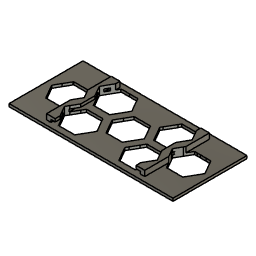
huine_solar_controller_mount (Autodesk Fusion 360 design; units mm, degrees)
Autodesk Fusion 360 part; units mm, degrees
sketch "Sketch1" plane through (0, 0, 0) normal (0, 0, 1) x (1, 0, 0)
  line L0 (0, 0) -> (-152, 0)
  line L1 (-152, 0) -> (-152, 68.58)
  line L2 (-152, 68.58) -> (0, 68.58)
  line L3 (0, 68.58) -> (0, 0)
  dimension "d1" = 152
  dimension "d2" = 68.58
  constraint horizontal L0
  constraint vertical L1
  constraint horizontal L2
  constraint vertical L3
  constraint coincident L0.start L3.end
  measures "d1" distance of L0.start L0.end
  measures "d2" distance of L0.start L2.end
extrude "Extrude1" add sketch "Sketch1" along normal blind 2.5
sketch "Sketch2" plane through (0, 0, 2.5) normal (0, 0, 1) x (-1, 0, 0)
  line L0 (0, -68.58) -> (152, -68.58)
  line L1 (152, -68.58) -> (152, 0)
  line L2 (152, 0) -> (0, 0)
  line L3 (0, 0) -> (0, -68.58)
  line L4 (76, -68.58) -> (76, 0) construction
  line L5 (152, -34.29) -> (0, -34.29) construction
  line L6 (117, -11.54) -> (35, -11.54) construction
  line L7 (35, -11.54) -> (35, -57.04) construction
  line L8 (35, -57.04) -> (117, -57.04) construction
  line L9 (117, -57.04) -> (117, -11.54) construction
  line L10 (117, -11.54) -> (35, -57.04) construction
  line L11 (35, -11.54) -> (117, -57.04) construction
  line L12 (113.5, -4.29) -> (120.5, -4.29)
  line L13 (120.5, -4.29) -> (120.5, -64.29)
  line L14 (120.5, -64.29) -> (113.5, -64.29)
  line L15 (113.5, -64.29) -> (113.5, -4.29)
  line L16 (113.5, -4.29) -> (120.5, -64.29) construction
  line L17 (120.5, -4.29) -> (113.5, -64.29) construction
  line L18 (31.5, -64.29) -> (38.5, -64.29)
  line L19 (38.5, -64.29) -> (38.5, -4.29)
  line L20 (31.5, -4.29) -> (31.5, -64.29)
  line L21 (38.5, -4.29) -> (31.5, -4.29)
  point P0 (76, -34.29)
  point P1 (117, -34.29)
  dimension "d5" = 82
  dimension "d6" = 45.5
  dimension "d7" = 7
  dimension "d8" = 60
  constraint midpoint L0 L4.start
  constraint midpoint L2 L4.end
  constraint midpoint L1 L5.start
  constraint midpoint L3 L5.end
  constraint horizontal L6
  constraint perpendicular L6 L7
  constraint parallel L6 L8
  constraint parallel L7 L9
  constraint coincident L10 P0
  constraint coincident L11 P0
  constraint midpoint L5 P0
  constraint horizontal L12
  constraint perpendicular L12 L13
  constraint parallel L12 L14
  constraint parallel L13 L15
  constraint coincident L16 P1
  constraint coincident L17 P1
  constraint midpoint L9 P1
  constraint symmetric L4 L12.start L19.end
  constraint symmetric L4 L12.end L20.start
  constraint symmetric L4 L13.end L18.start
  constraint symmetric L4 L14.end L18.end
  measures "d5" distance of L7.end L8.end
  measures "d6" distance of L6.end L7.end
  measures "d7" distance of L13.end L14.end
  measures "d8" distance of L12.end L13.end
extrude "Extrude2" add sketch "Sketch2" along normal blind 5 contours L12 L13 L14 L15 | L18 L19 L20 L21
sketch "Sketch4" plane through (-113.5, 0, 0) normal (1, 0, 0) x (0, 1, 0)
  line L0 (4.29, 2.5) -> (64.29, 2.5)
  line L1 (64.29, 2.5) -> (64.29, 7.5)
  line L2 (64.29, 7.5) -> (4.29, 7.5)
  line L3 (4.29, 7.5) -> (4.29, 2.5)
  line L4 (4.29, 2.5) -> (57.29, 2.5)
  line L5 (57.29, 2.5) -> (57.29, 4.8)
  line L6 (57.29, 4.8) -> (4.29, 4.8)
  line L7 (4.29, 4.8) -> (4.29, 2.5)
  dimension "d11" = 53
  dimension "d12" = 2.3
  constraint horizontal L4
  constraint vertical L5
  constraint horizontal L6
  constraint vertical L7
  constraint coincident L0.start L3.end
  measures "d11" distance of L0.start L4.end
  measures "d12" distance of L0.start L6.end
sketch "Sketch5" plane through (-38.5, 0, 0) normal (-1, 0, 0) x (0, -1, 0)
  line L0 (-64.29, 2.5) -> (-4.29, 2.5)
  line L1 (-4.29, 2.5) -> (-4.29, 7.5)
  line L2 (-4.29, 7.5) -> (-64.29, 7.5)
  line L3 (-64.29, 7.5) -> (-64.29, 2.5)
  line L4 (-4.29, 2.5) -> (-57.29, 2.5)
  line L5 (-57.29, 2.5) -> (-57.29, 4.8)
  line L6 (-57.29, 4.8) -> (-4.29, 4.8)
  line L7 (-4.29, 4.8) -> (-4.29, 2.5)
  dimension "d13" = 53
  dimension "d14" = 2.3
  constraint horizontal L4
  constraint vertical L5
  constraint horizontal L6
  constraint vertical L7
  constraint coincident L0.end L1.start
  measures "d13" distance of L0.end L4.end
  measures "d14" distance of L0.end L6.end
extrude "Extrude3" cut sketch "Sketch4" against normal blind 3.95 contours L0 L3 L4 L5 L6 L7
extrude "Extrude4" cut sketch "Sketch5" against normal blind 3.95 contours L0 L1 L4 L5 L6 L7
extrude "Extrude5" add 1 faces at (-31.5, 24.29, 4.1667) along direction (1, 0, 0) blind 1
move_face "OffsetFaces1" offset 1 1 faces at (-120.5, 24.29, 5.8333)
fillet "Fillet1" [suppressed]
sketch "Sketch6" plane through (0, 0, 0) normal (0, 0, -1) x (1, 0, 0)
  spline S0 degree 3 poles (-145.338, 13.0972) (-145.6222, 12.6381) (-146.8027, 10.605) (-147.9614, 8.55) knots 0 0 0 0 1 1 1 1
  spline S1 degree 3 poles (-147.9614, 8.55) (-149.1419, 6.5168) (-150.6066, 3.959) (-151.2406, 2.8659) knots 0 0 0 0 1 1 1 1
  line L0 (-151.2406, 2.8659) -> (-152.3774, 0.8984)
  line L1 (-152.3774, 0.8984) -> (-156.1595, 0.8328)
  line L2 (-156.1595, 0.8328) -> (-159.9197, 0.7891)
  line L3 (-159.9197, 0.7891) -> (-159.9197, -2.2715)
  line L4 (-159.9197, -2.2715) -> (-159.9197, -5.3322)
  line L5 (-159.9197, -5.3322) -> (-156.1376, -5.3322)
  line L6 (-156.1376, -5.3322) -> (-152.3774, -5.3322)
  line L7 (-152.3774, -5.3322) -> (-151.4811, -6.9281)
  spline S2 degree 3 poles (-151.4811, -6.9281) (-151.0001, -7.7807) (-149.3168, -10.732) (-147.7428, -13.4428) knots 0 0 0 0 1 1 1 1
  line L8 (-147.7428, -13.4428) -> (-144.8789, -18.4054)
  line L9 (-144.8789, -18.4054) -> (-146.9995, -22.0782)
  spline S3 degree 3 poles (-146.9995, -22.0782) (-148.1581, -24.1113) (-149.8415, -27.0189) (-150.7378, -28.5492) knots 0 0 0 0 1 1 1 1
  line L10 (-150.7378, -28.5492) -> (-152.3556, -31.3475)
  line L11 (-152.3556, -31.3475) -> (-156.1376, -31.3475)
  line L12 (-156.1376, -31.3475) -> (-159.9197, -31.3475)
  line L13 (-159.9197, -31.3475) -> (-159.9197, -34.5174)
  line L14 (-159.9197, -34.5174) -> (-159.9197, -37.6874)
  line L15 (-159.9197, -37.6874) -> (-156.1376, -37.6874)
  line L16 (-156.1376, -37.6874) -> (-152.3774, -37.6874)
  line L17 (-152.3774, -37.6874) -> (-151.4592, -39.2833)
  spline S4 degree 3 poles (-151.4592, -39.2833) (-150.9783, -40.1359) (-149.3168, -43.0216) (-147.7865, -45.6669) knots 0 0 0 0 1 1 1 1
  spline S5 degree 3 poles (-147.7865, -45.6669) (-146.2562, -48.3121) (-144.9882, -50.5639) (-144.9882, -50.695) knots 0 0 0 0 1 1 1 1
  spline S6 degree 3 poles (-144.9882, -50.695) (-144.9882, -50.8043) (-146.1031, -52.8375) (-147.4586, -55.1767) knots 0 0 0 0 1 1 1 1
  spline S7 degree 3 poles (-147.4586, -55.1767) (-148.814, -57.5159) (-150.4536, -60.4016) (-151.1313, -61.5603) knots 0 0 0 0 1 1 1 1
  line L18 (-151.1313, -61.5603) -> (-152.3556, -63.7027)
  line L19 (-152.3556, -63.7027) -> (-156.1376, -63.7027)
  line L20 (-156.1376, -63.7027) -> (-159.9197, -63.7027)
  line L21 (-159.9197, -63.7027) -> (-159.9197, -66.8726)
  line L22 (-159.9197, -66.8726) -> (-159.9197, -70.0426)
  line L23 (-159.9197, -70.0426) -> (-156.0939, -70.0426)
  line L24 (-156.0939, -70.0426) -> (-152.29, -70.0426)
  line L25 (-152.29, -70.0426) -> (-151.9183, -70.7421)
  spline S8 degree 3 poles (-151.9183, -70.7421) (-151.7216, -71.1356) (-150.082, -74.0214) (-148.2674, -77.1257) knots 0 0 0 0 1 1 1 1
  spline S9 degree 3 poles (-148.2674, -77.1257) (-146.4529, -80.2519) (-144.9882, -82.9191) (-144.9882, -83.0284) knots 0 0 0 0 1 1 1 1
  spline S10 degree 3 poles (-144.9882, -83.0284) (-144.9882, -83.1595) (-146.0594, -85.0834) (-147.3274, -87.3132) knots 0 0 0 0 1 1 1 1
  spline S11 degree 3 poles (-147.3274, -87.3132) (-148.6172, -89.5431) (-150.2787, -92.407) (-151.022, -93.6968) knots 0 0 0 0 1 1 1 1
  line L26 (-151.022, -93.6968) -> (-152.3774, -96.0579)
  line L27 (-152.3774, -96.0579) -> (-156.1376, -96.0579)
  line L28 (-156.1376, -96.0579) -> (-159.9197, -96.0579)
  line L29 (-159.9197, -96.0579) -> (-159.9197, -99.2278)
  line L30 (-159.9197, -99.2278) -> (-159.9197, -102.3978)
  line L31 (-159.9197, -102.3978) -> (-156.1158, -102.3978)
  line L32 (-156.1158, -102.3978) -> (-152.3118, -102.3978)
  line L33 (-152.3118, -102.3978) -> (-151.2188, -104.2997)
  spline S12 degree 3 poles (-151.2188, -104.2997) (-150.6285, -105.3709) (-148.9452, -108.2785) (-147.5023, -110.7708) knots 0 0 0 0 1 1 1 1
  line L34 (-147.5023, -110.7708) -> (-144.8789, -115.318)
  line L35 (-144.8789, -115.318) -> (-147.7428, -120.2806)
  spline S13 degree 3 poles (-147.7428, -120.2806) (-149.3168, -123.0133) (-151.0001, -125.9646) (-151.4811, -126.8172) knots 0 0 0 0 1 1 1 1
  line L36 (-151.4811, -126.8172) -> (-152.3774, -128.4131)
  line L37 (-152.3774, -128.4131) -> (-156.1376, -128.4131)
  line L38 (-156.1376, -128.4131) -> (-159.9197, -128.4131)
  line L39 (-159.9197, -128.4131) -> (-159.9197, -131.4737)
  line L40 (-159.9197, -131.4737) -> (-159.9197, -134.5343)
  line L41 (-159.9197, -134.5343) -> (-156.1595, -134.5781)
  line L42 (-156.1595, -134.5781) -> (-152.3774, -134.6436)
  line L43 (-152.3774, -134.6436) -> (-150.9783, -137.0484)
  spline S14 degree 3 poles (-150.9783, -137.0484) (-150.2131, -138.3601) (-148.5298, -141.2677) (-147.2618, -143.4976) knots 0 0 0 0 1 1 1 1
  line L44 (-147.2618, -143.4976) -> (-144.9445, -147.542)
  line L45 (-144.9445, -147.542) -> (-131.9368, -147.542)
  line L46 (-131.9368, -147.542) -> (-118.951, -147.542)
  line L47 (-118.951, -147.542) -> (-115.6499, -141.858)
  spline S15 degree 3 poles (-115.6499, -141.858) (-113.8573, -138.7099) (-112.152, -135.7804) (-111.8897, -135.3432) knots 0 0 0 0 1 1 1 1
  line L48 (-111.8897, -135.3432) -> (-111.4088, -134.5343)
  line L49 (-111.4088, -134.5343) -> (-103.9977, -134.5343)
  spline S16 degree 3 poles (-103.9977, -134.5343) (-98.3136, -134.5343) (-96.521, -134.5999) (-96.368, -134.7967) knots 0 0 0 0 1 1 1 1
  spline S17 degree 3 poles (-96.368, -134.7967) (-96.2368, -134.9497) (-95.1874, -136.7424) (-94.0069, -138.7974) knots 0 0 0 0 1 1 1 1
  spline S18 degree 3 poles (-94.0069, -138.7974) (-92.8264, -140.8305) (-91.1868, -143.6725) (-90.356, -145.0935) knots 0 0 0 0 1 1 1 1
  line L50 (-90.356, -145.0935) -> (-88.8257, -147.6513)
  line L51 (-88.8257, -147.6513) -> (-75.9055, -147.6076)
  line L52 (-75.9055, -147.6076) -> (-63.0071, -147.542)
  line L53 (-63.0071, -147.542) -> (-59.2688, -141.0491)
  line L54 (-59.2688, -141.0491) -> (-55.5305, -134.5562)
  line L55 (-55.5305, -134.5562) -> (-48.0319, -134.5343)
  line L56 (-48.0319, -134.5343) -> (-40.5334, -134.5343)
  line L57 (-40.5334, -134.5343) -> (-40.0524, -135.3432)
  spline S19 degree 3 poles (-40.0524, -135.3432) (-39.7901, -135.7804) (-38.0849, -138.7099) (-36.2922, -141.858) knots 0 0 0 0 1 1 1 1
  line L58 (-36.2922, -141.858) -> (-32.9911, -147.542)
  line L59 (-32.9911, -147.542) -> (-20.0053, -147.542)
  line L60 (-20.0053, -147.542) -> (-7.0195, -147.542)
  line L61 (-7.0195, -147.542) -> (-4.3743, -142.9511)
  spline S20 degree 3 poles (-4.3743, -142.9511) (-2.9314, -140.4151) (-1.2481, -137.5294) (-0.6359, -136.5019) knots 0 0 0 0 1 1 1 1
  line L62 (-0.6359, -136.5019) -> (0.4572, -134.6436)
  line L63 (0.4572, -134.6436) -> (4.2174, -134.5781)
  line L64 (4.2174, -134.5781) -> (7.9776, -134.5343)
  line L65 (7.9776, -134.5343) -> (7.9776, -131.4737)
  line L66 (7.9776, -131.4737) -> (7.9776, -128.4131)
  line L67 (7.9776, -128.4131) -> (4.2174, -128.4131)
  line L68 (4.2174, -128.4131) -> (0.4353, -128.4131)
  line L69 (0.4353, -128.4131) -> (-0.0238, -127.5823)
  spline S21 degree 3 poles (-0.0238, -127.5823) (-0.2643, -127.1451) (-1.9476, -124.1938) (-3.784, -121.0457) knots 0 0 0 0 1 1 1 1
  line L70 (-3.784, -121.0457) -> (-7.0851, -115.2961)
  line L71 (-7.0851, -115.2961) -> (-5.205, -112.0825)
  spline S22 degree 3 poles (-5.205, -112.0825) (-4.1775, -110.2898) (-2.516, -107.4041) (-1.4885, -105.6114) knots 0 0 0 0 1 1 1 1
  line L72 (-1.4885, -105.6114) -> (0.3697, -102.3978)
  line L73 (0.3697, -102.3978) -> (4.1736, -102.3978)
  line L74 (4.1736, -102.3978) -> (7.9776, -102.3978)
  line L75 (7.9776, -102.3978) -> (7.9776, -99.2278)
  line L76 (7.9776, -99.2278) -> (7.9776, -96.0579)
  line L77 (7.9776, -96.0579) -> (4.1955, -96.0579)
  line L78 (4.1955, -96.0579) -> (0.4353, -96.0579)
  line L79 (0.4353, -96.0579) -> (-0.8108, -93.9373)
  spline S23 degree 3 poles (-0.8108, -93.9373) (-1.4667, -92.7568) (-3.1282, -89.871) (-4.4836, -87.5319) knots 0 0 0 0 1 1 1 1
  spline S24 degree 3 poles (-4.4836, -87.5319) (-5.839, -85.1927) (-6.9539, -83.1595) (-6.9539, -83.0502) knots 0 0 0 0 1 1 1 1
  spline S25 degree 3 poles (-6.9539, -83.0502) (-6.9539, -82.9191) (-5.9483, -81.0608) (-4.7022, -78.8965) knots 0 0 0 0 1 1 1 1
  spline S26 degree 3 poles (-4.7022, -78.8965) (-3.4561, -76.7322) (-1.8165, -73.8465) (-1.0294, -72.4911) knots 0 0 0 0 1 1 1 1
  line L80 (-1.0294, -72.4911) -> (0.3697, -70.0426)
  line L81 (0.3697, -70.0426) -> (4.1736, -70.0426)
  line L82 (4.1736, -70.0426) -> (7.9776, -70.0426)
  line L83 (7.9776, -70.0426) -> (7.9776, -66.8726)
  line L84 (7.9776, -66.8726) -> (7.9776, -63.7027)
  line L85 (7.9776, -63.7027) -> (4.1955, -63.7027)
  line L86 (4.1955, -63.7027) -> (0.4134, -63.7027)
  line L87 (0.4134, -63.7027) -> (-3.2812, -57.3191)
  spline S27 degree 3 poles (-3.2812, -57.3191) (-5.3143, -53.7994) (-6.9539, -50.8262) (-6.9539, -50.695) knots 0 0 0 0 1 1 1 1
  spline S28 degree 3 poles (-6.9539, -50.695) (-6.9539, -50.5857) (-6.0357, -48.9024) (-4.9208, -46.9786) knots 0 0 0 0 1 1 1 1
  spline S29 degree 3 poles (-4.9208, -46.9786) (-3.8277, -45.0547) (-2.1662, -42.169) (-1.2481, -40.5731) knots 0 0 0 0 1 1 1 1
  line L88 (-1.2481, -40.5731) -> (0.4134, -37.6874)
  line L89 (0.4134, -37.6874) -> (4.1955, -37.6874)
  line L90 (4.1955, -37.6874) -> (7.9776, -37.6874)
  line L91 (7.9776, -37.6874) -> (7.9776, -34.5174)
  line L92 (7.9776, -34.5174) -> (7.9776, -31.3475)
  line L93 (7.9776, -31.3475) -> (4.1736, -31.3475)
  line L94 (4.1736, -31.3475) -> (0.3916, -31.3475)
  line L95 (0.3916, -31.3475) -> (-3.1063, -25.27)
  spline S30 degree 3 poles (-3.1063, -25.27) (-5.0301, -21.947) (-6.7135, -19.0175) (-6.8228, -18.7771) knots 0 0 0 0 1 1 1 1
  spline S31 degree 3 poles (-6.8228, -18.7771) (-7.0195, -18.4054) (-6.626, -17.5965) (-4.4617, -13.8582) knots 0 0 0 0 1 1 1 1
  spline S32 degree 3 poles (-4.4617, -13.8582) (-3.0407, -11.3878) (-1.3574, -8.4584) (-0.7234, -7.3653) knots 0 0 0 0 1 1 1 1
  line L96 (-0.7234, -7.3653) -> (0.4353, -5.3322)
  line L97 (0.4353, -5.3322) -> (4.2174, -5.3322)
  line L98 (4.2174, -5.3322) -> (7.9776, -5.3322)
  line L99 (7.9776, -5.3322) -> (7.9776, -2.2715)
  line L100 (7.9776, -2.2715) -> (7.9776, 0.7891)
  line L101 (7.9776, 0.7891) -> (4.2174, 0.8328)
  line L102 (4.2174, 0.8328) -> (0.4353, 0.8984)
  line L103 (0.4353, 0.8984) -> (-0.9639, 3.3032)
  spline S33 degree 3 poles (-0.9639, 3.3032) (-1.729, 4.6367) (-3.4124, 7.5225) (-4.6803, 9.7524) knots 0 0 0 0 1 1 1 1
  line L104 (-4.6803, 9.7524) -> (-7.0195, 13.7968)
  line L105 (-7.0195, 13.7968) -> (-20.0053, 13.7968)
  line L106 (-20.0053, 13.7968) -> (-32.9911, 13.7968)
  line L107 (-32.9911, 13.7968) -> (-34.7619, 10.7361)
  spline S34 degree 3 poles (-34.7619, 10.7361) (-35.7457, 9.0528) (-37.429, 6.1452) (-38.5003, 4.2869) knots 0 0 0 0 1 1 1 1
  line L108 (-38.5003, 4.2869) -> (-40.4459, 0.8984)
  line L109 (-40.4459, 0.8984) -> (-47.9882, 0.8547)
  line L110 (-47.9882, 0.8547) -> (-55.5305, 0.7891)
  line L111 (-55.5305, 0.7891) -> (-56.6017, 2.7129)
  spline S35 degree 3 poles (-56.6017, 2.7129) (-57.1919, 3.7623) (-58.5255, 6.0359) (-59.5311, 7.7848) knots 0 0 0 0 1 1 1 1
  spline S36 degree 3 poles (-59.5311, 7.7848) (-61.5205, 11.1734) (-61.761, 11.5669) (-62.5043, 12.9223) knots 0 0 0 0 1 1 1 1
  line L112 (-62.5043, 12.9223) -> (-62.9853, 13.7968)
  line L113 (-62.9853, 13.7968) -> (-75.9711, 13.7968)
  line L114 (-75.9711, 13.7968) -> (-88.9569, 13.7968)
  line L115 (-88.9569, 13.7968) -> (-92.6952, 7.3476)
  line L116 (-92.6952, 7.3476) -> (-96.4335, 0.8984)
  line L117 (-96.4335, 0.8984) -> (-103.9102, 0.8328)
  line L118 (-103.9102, 0.8328) -> (-111.4088, 0.7891)
  line L119 (-111.4088, 0.7891) -> (-111.8897, 1.598)
  spline S37 degree 3 poles (-111.8897, 1.598) (-112.152, 2.0352) (-113.8573, 4.9647) (-115.6499, 8.1127) knots 0 0 0 0 1 1 1 1
  line L120 (-115.6499, 8.1127) -> (-118.951, 13.7968)
  line L121 (-118.951, 13.7968) -> (-131.8931, 13.8623)
  line L122 (-131.8931, 13.8623) -> (-144.8352, 13.9061)
  line L123 (-144.8352, 13.9061) -> (-145.338, 13.0972)
  spline S38 degree 3 poles (-124.329, 10.5831) (-124.1978, 10.4301) (-122.4926, 7.4787) (-120.5032, 4.0246) knots 0 0 0 0 1 1 1 1
  line L124 (-120.5032, 4.0246) -> (-116.896, -2.2715)
  line L125 (-116.896, -2.2715) -> (-119.6287, -7.0155)
  spline S39 degree 3 poles (-119.6287, -7.0155) (-121.159, -9.6389) (-122.8424, -12.5465) (-123.3889, -13.4865) knots 0 0 0 0 1 1 1 1
  line L126 (-123.3889, -13.4865) -> (-124.3946, -15.1918)
  line L127 (-124.3946, -15.1918) -> (-129.2041, -15.1918)
  spline S40 degree 3 poles (-129.2041, -15.1918) (-131.8494, -15.1918) (-135.2598, -15.1918) (-136.7901, -15.1699) knots 0 0 0 0 1 1 1 1
  line L128 (-136.7901, -15.1699) -> (-139.5665, -15.1699)
  line L129 (-139.5665, -15.1699) -> (-141.1406, -12.3716)
  spline S41 degree 3 poles (-141.1406, -12.3716) (-142.015, -10.8413) (-143.6984, -7.9556) (-144.8789, -5.9224) knots 0 0 0 0 1 1 1 1
  line L130 (-144.8789, -5.9224) -> (-146.9995, -2.2715)
  line L131 (-146.9995, -2.2715) -> (-145.7752, -0.1291)
  spline S42 degree 3 poles (-145.7752, -0.1291) (-145.1194, 1.0296) (-143.8951, 3.1283) (-143.0862, 4.5056) knots 0 0 0 0 1 1 1 1
  spline S43 degree 3 poles (-143.0862, 4.5056) (-142.2774, 5.8828) (-141.3154, 7.5662) (-140.9438, 8.222) knots 0 0 0 0 1 1 1 1
  spline S44 degree 3 poles (-140.9438, 8.222) (-140.594, 8.8779) (-140.1131, 9.7524) (-139.8944, 10.124) knots 0 0 0 0 1 1 1 1
  line L132 (-139.8944, 10.124) -> (-139.4791, 10.8454)
  line L133 (-139.4791, 10.8454) -> (-132.0243, 10.8454)
  spline S45 degree 3 poles (-132.0243, 10.8454) (-126.3184, 10.8454) (-124.5039, 10.7798) (-124.329, 10.5831) knots 0 0 0 0 1 1 1 1
  spline S46 degree 3 poles (-67.4888, 9.0965) (-66.9422, 8.2002) (-65.2589, 5.2707) (-63.7286, 2.5817) knots 0 0 0 0 1 1 1 1
  line L134 (-63.7286, 2.5817) -> (-60.9303, -2.2715)
  line L135 (-60.9303, -2.2715) -> (-64.603, -8.6333)
  spline S47 degree 3 poles (-64.603, -8.6333) (-66.6362, -12.1311) (-68.3414, -15.0387) (-68.4069, -15.1043) knots 0 0 0 0 1 1 1 1
  spline S48 degree 3 poles (-68.4069, -15.1043) (-68.5381, -15.2355) (-68.3195, -15.2355) (-76.8674, -15.1918) knots 0 0 0 0 1 1 1 1
  line L136 (-76.8674, -15.1918) -> (-83.5789, -15.1699)
  line L137 (-83.5789, -15.1699) -> (-84.672, -13.2461)
  spline S49 degree 3 poles (-84.672, -13.2461) (-85.2841, -12.1967) (-86.9456, -9.2891) (-88.3885, -6.7969) knots 0 0 0 0 1 1 1 1
  line L138 (-88.3885, -6.7969) -> (-91.0337, -2.2497)
  line L139 (-91.0337, -2.2497) -> (-88.6727, 1.8384)
  spline S50 degree 3 poles (-88.6727, 1.8384) (-87.3828, 4.0902) (-85.6995, 7.0415) (-84.9125, 8.3751) knots 0 0 0 0 1 1 1 1
  line L140 (-84.9125, 8.3751) -> (-83.5133, 10.8236)
  line L141 (-83.5133, 10.8236) -> (-75.9711, 10.7798)
  line L142 (-75.9711, 10.7798) -> (-68.4507, 10.7361)
  line L143 (-68.4507, 10.7361) -> (-67.4888, 9.0965)
  spline S51 degree 3 poles (-10.9546, 8.1565) (-10.1239, 6.6917) (-8.4187, 3.7404) (-7.1944, 1.6198) knots 0 0 0 0 1 1 1 1
  line L144 (-7.1944, 1.6198) -> (-4.9427, -2.2497)
  line L145 (-4.9427, -2.2497) -> (-8.7029, -8.7207)
  line L146 (-8.7029, -8.7207) -> (-12.4631, -15.1918)
  line L147 (-12.4631, -15.1918) -> (-20.0053, -15.1918)
  line L148 (-20.0053, -15.1918) -> (-27.5476, -15.1918)
  line L149 (-27.5476, -15.1918) -> (-28.5095, -13.5959)
  spline S52 degree 3 poles (-28.5095, -13.5959) (-29.0342, -12.7214) (-30.7175, -9.8138) (-32.2697, -7.1248) knots 0 0 0 0 1 1 1 1
  line L150 (-32.2697, -7.1248) -> (-35.068, -2.2278)
  line L151 (-35.068, -2.2278) -> (-31.4389, 4.0246)
  spline S53 degree 3 poles (-31.4389, 4.0246) (-29.4495, 7.4787) (-27.7225, 10.4301) (-27.6132, 10.5831) knots 0 0 0 0 1 1 1 1
  spline S54 degree 3 poles (-27.6132, 10.5831) (-27.4383, 10.7798) (-25.6238, 10.8454) (-19.9179, 10.8454) knots 0 0 0 0 1 1 1 1
  line L152 (-19.9179, 10.8454) -> (-12.4631, 10.8236)
  line L153 (-12.4631, 10.8236) -> (-10.9546, 8.1565)
  spline S55 degree 3 poles (-95.7777, -6.4908) (-95.4279, -7.103) (-93.7664, -9.9887) (-92.0831, -12.8744) knots 0 0 0 0 1 1 1 1
  spline S56 degree 3 poles (-92.0831, -12.8744) (-90.3997, -15.7602) (-89.0225, -18.2961) (-89.0443, -18.5147) knots 0 0 0 0 1 1 1 1
  spline S57 degree 3 poles (-89.0443, -18.5147) (-89.0443, -18.7552) (-89.2411, -19.1924) (-89.4597, -19.4985) knots 0 0 0 0 1 1 1 1
  spline S58 degree 3 poles (-89.4597, -19.4985) (-89.6783, -19.8264) (-89.9625, -20.2855) (-90.0937, -20.526) knots 0 0 0 0 1 1 1 1
  spline S59 degree 3 poles (-90.0937, -20.526) (-90.2248, -20.7665) (-90.8588, -21.8377) (-91.4928, -22.9308) knots 0 0 0 0 1 1 1 1
  spline S60 degree 3 poles (-91.4928, -22.9308) (-92.1268, -24.002) (-93.4822, -26.3412) (-94.5097, -28.112) knots 0 0 0 0 1 1 1 1
  line L154 (-94.5097, -28.112) -> (-96.3461, -31.3475)
  line L155 (-96.3461, -31.3475) -> (-103.9539, -31.3475)
  line L156 (-103.9539, -31.3475) -> (-111.5399, -31.3475)
  line L157 (-111.5399, -31.3475) -> (-113.4637, -28.0027)
  spline S61 degree 3 poles (-113.4637, -28.0027) (-114.5131, -26.1882) (-116.1964, -23.2587) (-117.2021, -21.5535) knots 0 0 0 0 1 1 1 1
  line L158 (-117.2021, -21.5535) -> (-119.0166, -18.4054)
  line L159 (-119.0166, -18.4054) -> (-116.6774, -14.3392)
  spline S62 degree 3 poles (-116.6774, -14.3392) (-115.3657, -12.0874) (-113.6824, -9.1579) (-112.8953, -7.8025) knots 0 0 0 0 1 1 1 1
  line L160 (-112.8953, -7.8025) -> (-111.4962, -5.354)
  line L161 (-111.4962, -5.354) -> (-103.9539, -5.3322)
  line L162 (-103.9539, -5.3322) -> (-96.4117, -5.3322)
  line L163 (-96.4117, -5.3322) -> (-95.7777, -6.4908)
  spline S63 degree 3 poles (-38.3691, -8.9831) (-37.2323, -10.9725) (-35.5271, -13.9238) (-34.6089, -15.5197) knots 0 0 0 0 1 1 1 1
  line L164 (-34.6089, -15.5197) -> (-32.9255, -18.4054)
  line L165 (-32.9255, -18.4054) -> (-34.7401, -21.5535)
  spline S64 degree 3 poles (-34.7401, -21.5535) (-35.7457, -23.2587) (-37.429, -26.1882) (-38.4784, -28.0027) knots 0 0 0 0 1 1 1 1
  line L166 (-38.4784, -28.0027) -> (-40.4241, -31.3475)
  line L167 (-40.4241, -31.3475) -> (-48.0101, -31.3475)
  line L168 (-48.0101, -31.3475) -> (-55.596, -31.3475)
  line L169 (-55.596, -31.3475) -> (-57.8915, -27.3468)
  spline S65 degree 3 poles (-57.8915, -27.3468) (-59.1595, -25.1607) (-60.8428, -22.2531) (-61.6298, -20.8758) knots 0 0 0 0 1 1 1 1
  line L170 (-61.6298, -20.8758) -> (-63.0727, -18.4054)
  line L171 (-63.0727, -18.4054) -> (-60.2088, -13.4428)
  spline S66 degree 3 poles (-60.2088, -13.4428) (-58.6348, -10.732) (-56.9296, -7.7807) (-56.4268, -6.9281) knots 0 0 0 0 1 1 1 1
  line L172 (-56.4268, -6.9281) -> (-55.5305, -5.3322)
  line L173 (-55.5305, -5.3322) -> (-47.9882, -5.3322)
  line L174 (-47.9882, -5.3322) -> (-40.4459, -5.354)
  line L175 (-40.4459, -5.354) -> (-38.3691, -8.9831)
  spline S67 degree 3 poles (-121.2246, -27.0189) (-119.4757, -30.0577) (-117.7923, -32.9871) (-117.4644, -33.5555) knots 0 0 0 0 1 1 1 1
  line L176 (-117.4644, -33.5555) -> (-116.8742, -34.5612)
  line L177 (-116.8742, -34.5612) -> (-119.0822, -38.3651)
  spline S68 degree 3 poles (-119.0822, -38.3651) (-120.2846, -40.4638) (-121.9679, -43.3714) (-122.8424, -44.8361) knots 0 0 0 0 1 1 1 1
  line L178 (-122.8424, -44.8361) -> (-124.3946, -47.5251)
  line L179 (-124.3946, -47.5251) -> (-131.9805, -47.5251)
  line L180 (-131.9805, -47.5251) -> (-139.5665, -47.5251)
  line L181 (-139.5665, -47.5251) -> (-139.8289, -47.0223)
  spline S69 degree 3 poles (-139.8289, -47.0223) (-139.96, -46.7599) (-141.6215, -43.8961) (-143.4798, -40.6605) knots 0 0 0 0 1 1 1 1
  spline S70 degree 3 poles (-143.4798, -40.6605) (-145.338, -37.425) (-146.8683, -34.6705) (-146.8683, -34.5393) knots 0 0 0 0 1 1 1 1
  spline S71 degree 3 poles (-146.8683, -34.5393) (-146.8683, -34.4081) (-145.6878, -32.2875) (-144.2668, -29.8172) knots 0 0 0 0 1 1 1 1
  spline S72 degree 3 poles (-144.2668, -29.8172) (-142.8239, -27.3468) (-141.1624, -24.4829) (-140.5722, -23.4336) knots 0 0 0 0 1 1 1 1
  line L182 (-140.5722, -23.4336) -> (-139.4791, -21.5098)
  line L183 (-139.4791, -21.5098) -> (-131.9368, -21.5098)
  line L184 (-131.9368, -21.5098) -> (-124.3946, -21.5098)
  line L185 (-124.3946, -21.5098) -> (-121.2246, -27.0189)
  spline S73 degree 3 poles (-67.2046, -23.6522) (-66.5268, -24.8109) (-64.8654, -27.6966) (-63.5099, -30.0358) knots 0 0 0 0 1 1 1 1
  spline S74 degree 3 poles (-63.5099, -30.0358) (-62.1545, -32.375) (-61.0396, -34.4081) (-61.0396, -34.5174) knots 0 0 0 0 1 1 1 1
  spline S75 degree 3 poles (-61.0396, -34.5174) (-61.0396, -34.6486) (-62.7011, -37.6218) (-64.7342, -41.1415) knots 0 0 0 0 1 1 1 1
  line L186 (-64.7342, -41.1415) -> (-68.4288, -47.5251)
  line L187 (-68.4288, -47.5251) -> (-75.9929, -47.5251)
  line L188 (-75.9929, -47.5251) -> (-83.5571, -47.5251)
  line L189 (-83.5571, -47.5251) -> (-87.1861, -41.2289)
  spline S76 degree 3 poles (-87.1861, -41.2289) (-89.1755, -37.7748) (-90.837, -34.8454) (-90.8807, -34.6923) knots 0 0 0 0 1 1 1 1
  spline S77 degree 3 poles (-90.8807, -34.6923) (-90.9244, -34.5612) (-89.2629, -31.5442) (-87.2298, -27.9808) knots 0 0 0 0 1 1 1 1
  line L190 (-87.2298, -27.9808) -> (-83.5133, -21.5098)
  line L191 (-83.5133, -21.5098) -> (-75.9711, -21.5098)
  line L192 (-75.9711, -21.5098) -> (-68.4288, -21.5098)
  line L193 (-68.4288, -21.5098) -> (-67.2046, -23.6522)
  spline S78 degree 3 poles (-11.37, -23.4336) (-10.7797, -24.4829) (-9.1182, -27.3468) (-7.6754, -29.8172) knots 0 0 0 0 1 1 1 1
  spline S79 degree 3 poles (-7.6754, -29.8172) (-6.2544, -32.2875) (-5.0738, -34.4081) (-5.0738, -34.5393) knots 0 0 0 0 1 1 1 1
  spline S80 degree 3 poles (-5.0738, -34.5393) (-5.0738, -34.6923) (-6.1451, -36.6599) (-7.4786, -38.9116) knots 0 0 0 0 1 1 1 1
  spline S81 degree 3 poles (-7.4786, -38.9116) (-8.7903, -41.1852) (-10.4518, -44.0491) (-11.1514, -45.2733) knots 0 0 0 0 1 1 1 1
  line L194 (-11.1514, -45.2733) -> (-12.4412, -47.5251)
  line L195 (-12.4412, -47.5251) -> (-16.9228, -47.547)
  spline S82 degree 3 poles (-16.9228, -47.547) (-19.3932, -47.547) (-21.7105, -47.5688) (-22.0822, -47.5688) knots 0 0 0 0 1 1 1 1
  spline S83 degree 3 poles (-22.0822, -47.5688) (-22.432, -47.5688) (-23.8311, -47.5688) (-25.1647, -47.547) knots 0 0 0 0 1 1 1 1
  line L196 (-25.1647, -47.547) -> (-27.5694, -47.5251)
  line L197 (-27.5694, -47.5251) -> (-31.3296, -41.0322)
  line L198 (-31.3296, -41.0322) -> (-35.0898, -34.5612)
  line L199 (-35.0898, -34.5612) -> (-33.4939, -31.8066)
  spline S84 degree 3 poles (-33.4939, -31.8066) (-32.5976, -30.2981) (-30.9143, -27.3468) (-29.7119, -25.27) knots 0 0 0 0 1 1 1 1
  line L200 (-29.7119, -25.27) -> (-27.5476, -21.5098)
  line L201 (-27.5476, -21.5098) -> (-20.0053, -21.5098)
  line L202 (-20.0053, -21.5098) -> (-12.4631, -21.5098)
  line L203 (-12.4631, -21.5098) -> (-11.37, -23.4336)
  spline S85 degree 3 poles (-94.9907, -40.1577) (-94.2255, -41.4913) (-92.564, -44.377) (-91.2961, -46.5413) knots 0 0 0 0 1 1 1 1
  spline S86 degree 3 poles (-91.2961, -46.5413) (-90.0281, -48.7056) (-89.0225, -50.6513) (-89.0225, -50.8481) knots 0 0 0 0 1 1 1 1
  spline S87 degree 3 poles (-89.0225, -50.8481) (-89.0443, -51.0448) (-89.2629, -51.5039) (-89.4815, -51.8318) knots 0 0 0 0 1 1 1 1
  spline S88 degree 3 poles (-89.4815, -51.8318) (-89.9188, -52.444) (-92.6952, -57.2098) (-95.1, -61.4509) knots 0 0 0 0 1 1 1 1
  line L204 (-95.1, -61.4509) -> (-96.368, -63.7027)
  line L205 (-96.368, -63.7027) -> (-103.9321, -63.7027)
  spline S89 degree 3 poles (-103.9321, -63.7027) (-110.9278, -63.7027) (-111.5181, -63.6808) (-111.7367, -63.3092) knots 0 0 0 0 1 1 1 1
  spline S90 degree 3 poles (-111.7367, -63.3092) (-112.8298, -61.5821) (-118.8854, -50.8699) (-118.8854, -50.695) knots 0 0 0 0 1 1 1 1
  spline S91 degree 3 poles (-118.8854, -50.695) (-118.8854, -50.5639) (-117.4207, -47.9623) (-115.6499, -44.9017) knots 0 0 0 0 1 1 1 1
  spline S92 degree 3 poles (-115.6499, -44.9017) (-113.8791, -41.8411) (-112.2176, -38.9553) (-111.9553, -38.5181) knots 0 0 0 0 1 1 1 1
  line L206 (-111.9553, -38.5181) -> (-111.4962, -37.6874)
  line L207 (-111.4962, -37.6874) -> (-103.9539, -37.6874)
  line L208 (-103.9539, -37.6874) -> (-96.4117, -37.6874)
  line L209 (-96.4117, -37.6874) -> (-94.9907, -40.1577)
  spline S93 degree 3 poles (-39.5496, -39.2833) (-39.0468, -40.1359) (-37.3853, -43.0216) (-35.855, -45.6669) knots 0 0 0 0 1 1 1 1
  spline S94 degree 3 poles (-35.855, -45.6669) (-34.3247, -48.3121) (-33.0567, -50.5639) (-33.0567, -50.695) knots 0 0 0 0 1 1 1 1
  spline S95 degree 3 poles (-33.0567, -50.695) (-33.0567, -50.8043) (-34.7182, -53.7994) (-36.7513, -57.2972) knots 0 0 0 0 1 1 1 1
  line L210 (-36.7513, -57.2972) -> (-40.4241, -63.7027)
  line L211 (-40.4241, -63.7027) -> (-48.0101, -63.7027)
  line L212 (-48.0101, -63.7027) -> (-55.596, -63.7027)
  line L213 (-55.596, -63.7027) -> (-56.8422, -61.4509)
  spline S96 degree 3 poles (-56.8422, -61.4509) (-58.0227, -59.3741) (-59.1813, -57.3628) (-61.9578, -52.7063) knots 0 0 0 0 1 1 1 1
  line L214 (-61.9578, -52.7063) -> (-63.0946, -50.7825)
  line L215 (-63.0946, -50.7825) -> (-59.3125, -44.224)
  line L216 (-59.3125, -44.224) -> (-55.5305, -37.6874)
  line L217 (-55.5305, -37.6874) -> (-47.9882, -37.6874)
  line L218 (-47.9882, -37.6874) -> (-40.4459, -37.6874)
  line L219 (-40.4459, -37.6874) -> (-39.5496, -39.2833)
  spline S97 degree 3 poles (-120.6781, -60.2486) (-118.6668, -63.7683) (-117.0053, -66.7415) (-117.0053, -66.8726) knots 0 0 0 0 1 1 1 1
  spline S98 degree 3 poles (-117.0053, -66.8726) (-117.0053, -67.0475) (-119.0603, -70.6547) (-124.0448, -79.2682) knots 0 0 0 0 1 1 1 1
  line L220 (-124.0448, -79.2682) -> (-124.3946, -79.8803)
  line L221 (-124.3946, -79.8803) -> (-131.9587, -79.8803)
  line L222 (-131.9587, -79.8803) -> (-139.5009, -79.8803)
  line L223 (-139.5009, -79.8803) -> (-140.0256, -78.9402)
  spline S99 degree 3 poles (-140.0256, -78.9402) (-140.3098, -78.4374) (-141.9713, -75.5517) (-143.7202, -72.5566) knots 0 0 0 0 1 1 1 1
  spline S100 degree 3 poles (-143.7202, -72.5566) (-145.4473, -69.5397) (-146.8683, -66.9819) (-146.8683, -66.8726) knots 0 0 0 0 1 1 1 1
  spline S101 degree 3 poles (-146.8683, -66.8726) (-146.8683, -66.7415) (-145.4473, -64.1836) (-143.7202, -61.1886) knots 0 0 0 0 1 1 1 1
  spline S102 degree 3 poles (-143.7202, -61.1886) (-141.9713, -58.1717) (-140.3098, -55.3078) (-140.0256, -54.7831) knots 0 0 0 0 1 1 1 1
  line L224 (-140.0256, -54.7831) -> (-139.5009, -53.865)
  line L225 (-139.5009, -53.865) -> (-131.9368, -53.865)
  line L226 (-131.9368, -53.865) -> (-124.3727, -53.865)
  line L227 (-124.3727, -53.865) -> (-120.6781, -60.2486)
  spline S103 degree 3 poles (-67.6418, -55.2204) (-67.2046, -55.9855) (-65.5649, -58.8494) (-63.969, -61.604) knots 0 0 0 0 1 1 1 1
  spline S104 degree 3 poles (-63.969, -61.604) (-62.395, -64.3585) (-61.0614, -66.6759) (-61.0396, -66.7852) knots 0 0 0 0 1 1 1 1
  spline S105 degree 3 poles (-61.0396, -66.7852) (-61.0177, -66.8726) (-62.6573, -69.8458) (-64.7123, -73.4092) knots 0 0 0 0 1 1 1 1
  line L228 (-64.7123, -73.4092) -> (-68.4069, -79.8803)
  line L229 (-68.4069, -79.8803) -> (-76.0148, -79.8803)
  line L230 (-76.0148, -79.8803) -> (-83.6008, -79.8803)
  line L231 (-83.6008, -79.8803) -> (-83.9724, -79.1589)
  spline S106 degree 3 poles (-83.9724, -79.1589) (-84.1692, -78.7872) (-85.8088, -75.9015) (-87.6233, -72.7753) knots 0 0 0 0 1 1 1 1
  spline S107 degree 3 poles (-87.6233, -72.7753) (-89.4378, -69.6709) (-90.9026, -67.0038) (-90.9026, -66.8726) knots 0 0 0 0 1 1 1 1
  spline S108 degree 3 poles (-90.9026, -66.8726) (-90.9026, -66.7633) (-89.5471, -64.293) (-87.8857, -61.4072) knots 0 0 0 0 1 1 1 1
  spline S109 degree 3 poles (-87.8857, -61.4072) (-86.2242, -58.5215) (-84.5627, -55.6358) (-84.191, -55.0018) knots 0 0 0 0 1 1 1 1
  line L232 (-84.191, -55.0018) -> (-83.5352, -53.865)
  line L233 (-83.5352, -53.865) -> (-75.9711, -53.865)
  line L234 (-75.9711, -53.865) -> (-68.4069, -53.865)
  line L235 (-68.4069, -53.865) -> (-67.6418, -55.2204)
  spline S110 degree 3 poles (-11.37, -55.7669) (-10.7797, -56.8381) (-9.0964, -59.7457) (-7.6316, -62.2598) knots 0 0 0 0 1 1 1 1
  line L236 (-7.6316, -62.2598) -> (-4.9645, -66.8289)
  line L237 (-4.9645, -66.8289) -> (-5.6422, -68.0532)
  spline S111 degree 3 poles (-5.6422, -68.0532) (-6.0357, -68.7309) (-7.7191, -71.6822) (-9.4024, -74.5898) knots 0 0 0 0 1 1 1 1
  line L238 (-9.4024, -74.5898) -> (-12.4631, -79.8803)
  line L239 (-12.4631, -79.8803) -> (-20.0053, -79.8803)
  line L240 (-20.0053, -79.8803) -> (-27.5476, -79.8803)
  line L241 (-27.5476, -79.8803) -> (-27.8974, -79.2682)
  spline S112 degree 3 poles (-27.8974, -79.2682) (-28.0941, -78.9402) (-29.7556, -76.0764) (-31.592, -72.8846) knots 0 0 0 0 1 1 1 1
  spline S113 degree 3 poles (-31.592, -72.8846) (-33.4284, -69.6928) (-34.9368, -66.9819) (-34.9368, -66.8726) knots 0 0 0 0 1 1 1 1
  spline S114 degree 3 poles (-34.9368, -66.8726) (-34.9368, -66.7415) (-33.2753, -63.7683) (-31.2641, -60.2486) knots 0 0 0 0 1 1 1 1
  line L242 (-31.2641, -60.2486) -> (-27.5694, -53.865)
  line L243 (-27.5694, -53.865) -> (-20.0053, -53.865)
  line L244 (-20.0053, -53.865) -> (-12.4412, -53.865)
  line L245 (-12.4412, -53.865) -> (-11.37, -55.7669)
  spline S115 degree 3 poles (-95.1, -72.2724) (-94.4004, -73.5186) (-92.6952, -76.448) (-91.3179, -78.7872) knots 0 0 0 0 1 1 1 1
  spline S116 degree 3 poles (-91.3179, -78.7872) (-89.1755, -82.46) (-88.8694, -83.0939) (-89.088, -83.4656) knots 0 0 0 0 1 1 1 1
  spline S117 degree 3 poles (-89.088, -83.4656) (-89.2411, -83.6842) (-89.5253, -84.187) (-89.7439, -84.5587) knots 0 0 0 0 1 1 1 1
  spline S118 degree 3 poles (-89.7439, -84.5587) (-89.9406, -84.9303) (-90.8588, -86.4606) (-91.7333, -87.9691) knots 0 0 0 0 1 1 1 1
  spline S119 degree 3 poles (-91.7333, -87.9691) (-92.6296, -89.4775) (-94.0506, -91.9042) (-94.8814, -93.3689) knots 0 0 0 0 1 1 1 1
  line L246 (-94.8814, -93.3689) -> (-96.3898, -96.0579)
  line L247 (-96.3898, -96.0579) -> (-103.9539, -96.0579)
  line L248 (-103.9539, -96.0579) -> (-111.4962, -96.0579)
  line L249 (-111.4962, -96.0579) -> (-115.2783, -89.5213)
  line L250 (-115.2783, -89.5213) -> (-119.0385, -82.9846)
  line L251 (-119.0385, -82.9846) -> (-117.3333, -80.077)
  spline S120 degree 3 poles (-117.3333, -80.077) (-116.3932, -78.4593) (-114.688, -75.5517) (-113.5512, -73.5841) knots 0 0 0 0 1 1 1 1
  line L252 (-113.5512, -73.5841) -> (-111.4962, -70.0426)
  line L253 (-111.4962, -70.0426) -> (-103.9321, -70.0426)
  line L254 (-103.9321, -70.0426) -> (-96.368, -70.0426)
  line L255 (-96.368, -70.0426) -> (-95.1, -72.2724)
  spline S121 degree 3 poles (-39.7682, -71.1794) (-36.2266, -77.3006) (-33.1004, -82.766) (-33.0567, -82.9191) knots 0 0 0 0 1 1 1 1
  spline S122 degree 3 poles (-33.0567, -82.9191) (-33.0348, -83.0284) (-34.6745, -86.0234) (-36.7295, -89.5868) knots 0 0 0 0 1 1 1 1
  line L256 (-36.7295, -89.5868) -> (-40.4459, -96.0579)
  line L257 (-40.4459, -96.0579) -> (-47.9882, -96.0579)
  line L258 (-47.9882, -96.0579) -> (-55.5523, -96.0579)
  line L259 (-55.5523, -96.0579) -> (-57.8259, -92.0572)
  spline S123 degree 3 poles (-57.8259, -92.0572) (-59.072, -89.871) (-60.4493, -87.4881) (-60.8866, -86.7667) knots 0 0 0 0 1 1 1 1
  spline S124 degree 3 poles (-60.8866, -86.7667) (-61.3238, -86.0453) (-61.9796, -84.9085) (-62.3731, -84.2308) knots 0 0 0 0 1 1 1 1
  line L260 (-62.3731, -84.2308) -> (-63.0727, -83.0065)
  line L261 (-63.0727, -83.0065) -> (-61.0396, -79.5305)
  spline S125 degree 3 poles (-61.0396, -79.5305) (-59.9246, -77.6285) (-58.2413, -74.6991) (-57.3012, -73.0376) knots 0 0 0 0 1 1 1 1
  line L262 (-57.3012, -73.0376) -> (-55.596, -70.0426)
  line L263 (-55.596, -70.0426) -> (-48.0101, -70.0426)
  line L264 (-48.0101, -70.0426) -> (-40.4241, -70.0426)
  line L265 (-40.4241, -70.0426) -> (-39.7682, -71.1794)
  spline S126 degree 3 poles (-124.1322, -86.6137) (-122.9517, -88.5375) (-117.0053, -99.0311) (-117.0053, -99.206) knots 0 0 0 0 1 1 1 1
  spline S127 degree 3 poles (-117.0053, -99.206) (-117.0053, -99.3371) (-117.7923, -100.78) (-118.7324, -102.3978) knots 0 0 0 0 1 1 1 1
  spline S128 degree 3 poles (-118.7324, -102.3978) (-119.6943, -104.0155) (-121.3558, -106.9013) (-122.427, -108.7813) knots 0 0 0 0 1 1 1 1
  line L266 (-122.427, -108.7813) -> (-124.3946, -112.2355)
  line L267 (-124.3946, -112.2355) -> (-131.9368, -112.2355)
  line L268 (-131.9368, -112.2355) -> (-139.4791, -112.2355)
  line L269 (-139.4791, -112.2355) -> (-140.3754, -110.6396)
  spline S129 degree 3 poles (-140.3754, -110.6396) (-140.8782, -109.787) (-142.5616, -106.8357) (-144.1575, -104.1248) knots 0 0 0 0 1 1 1 1
  line L270 (-144.1575, -104.1248) -> (-147.0213, -99.1622)
  line L271 (-147.0213, -99.1622) -> (-144.551, -94.9429)
  spline S130 degree 3 poles (-144.551, -94.9429) (-143.1955, -92.6038) (-141.5122, -89.6962) (-140.8126, -88.4719) knots 0 0 0 0 1 1 1 1
  line L272 (-140.8126, -88.4719) -> (-139.5447, -86.2202)
  line L273 (-139.5447, -86.2202) -> (-132.4178, -86.1764)
  spline S131 degree 3 poles (-132.4178, -86.1764) (-128.4827, -86.1327) (-125.0723, -86.1327) (-124.8099, -86.1764) knots 0 0 0 0 1 1 1 1
  spline S132 degree 3 poles (-124.8099, -86.1764) (-124.5694, -86.2202) (-124.2634, -86.4169) (-124.1322, -86.6137) knots 0 0 0 0 1 1 1 1
  spline S133 degree 3 poles (-12.2882, -86.5044) (-12.2007, -86.6574) (-10.4955, -89.565) (-8.528, -92.9973) knots 0 0 0 0 1 1 1 1
  line L274 (-8.528, -92.9973) -> (-4.9427, -99.2278)
  line L275 (-4.9427, -99.2278) -> (-5.358, -99.8837)
  spline S134 degree 3 poles (-5.358, -99.8837) (-5.8827, -100.78) (-11.0202, -109.6558) (-11.8291, -111.0768) knots 0 0 0 0 1 1 1 1
  line L276 (-11.8291, -111.0768) -> (-12.4631, -112.2355)
  line L277 (-12.4631, -112.2355) -> (-20.0053, -112.2355)
  line L278 (-20.0053, -112.2355) -> (-27.5476, -112.2355)
  line L279 (-27.5476, -112.2355) -> (-29.7119, -108.4534)
  spline S135 degree 3 poles (-29.7119, -108.4534) (-30.9143, -106.3984) (-32.6195, -103.4471) (-33.4939, -101.9168) knots 0 0 0 0 1 1 1 1
  line L280 (-33.4939, -101.9168) -> (-35.1117, -99.1404)
  line L281 (-35.1117, -99.1404) -> (-34.587, -98.3096)
  spline S136 degree 3 poles (-34.587, -98.3096) (-34.3028, -97.8505) (-32.6632, -95.0085) (-30.9361, -92.0135) knots 0 0 0 0 1 1 1 1
  spline S137 degree 3 poles (-30.9361, -92.0135) (-29.2091, -88.9966) (-27.7443, -86.4388) (-27.635, -86.3295) knots 0 0 0 0 1 1 1 1
  spline S138 degree 3 poles (-27.635, -86.3295) (-27.3945, -86.0015) (-12.5068, -86.1546) (-12.2882, -86.5044) knots 0 0 0 0 1 1 1 1
  spline S139 degree 3 poles (-66.4175, -89.6524) (-65.3245, -91.5544) (-63.6411, -94.462) (-62.6792, -96.1235) knots 0 0 0 0 1 1 1 1
  line L282 (-62.6792, -96.1235) -> (-60.9521, -99.1622)
  line L283 (-60.9521, -99.1622) -> (-62.2857, -101.5014)
  spline S140 degree 3 poles (-62.2857, -101.5014) (-63.0071, -102.8131) (-64.6905, -105.7426) (-66.024, -108.0381) knots 0 0 0 0 1 1 1 1
  line L284 (-66.024, -108.0381) -> (-68.4288, -112.2355)
  line L285 (-68.4288, -112.2355) -> (-75.9711, -112.2355)
  line L286 (-75.9711, -112.2355) -> (-83.5133, -112.2355)
  line L287 (-83.5133, -112.2355) -> (-87.2954, -105.6551)
  spline S141 degree 3 poles (-87.2954, -105.6551) (-89.9188, -101.1079) (-91.0119, -99.0092) (-90.8807, -98.8343) knots 0 0 0 0 1 1 1 1
  spline S142 degree 3 poles (-90.8807, -98.8343) (-90.6839, -98.6157) (-88.6727, -95.1178) (-84.672, -88.1221) knots 0 0 0 0 1 1 1 1
  line L288 (-84.672, -88.1221) -> (-83.5789, -86.2202)
  line L289 (-83.5789, -86.2202) -> (-75.9711, -86.2202)
  line L290 (-75.9711, -86.2202) -> (-68.3851, -86.2202)
  line L291 (-68.3851, -86.2202) -> (-66.4175, -89.6524)
  spline S143 degree 3 poles (-93.5478, -107.251) (-92.0175, -109.94) (-90.3342, -112.8257) (-89.8095, -113.7002) knots 0 0 0 0 1 1 1 1
  line L292 (-89.8095, -113.7002) -> (-88.8694, -115.2743)
  line L293 (-88.8694, -115.2743) -> (-92.6296, -121.8327)
  line L294 (-92.6296, -121.8327) -> (-96.4117, -128.4131)
  line L295 (-96.4117, -128.4131) -> (-103.9539, -128.4131)
  line L296 (-103.9539, -128.4131) -> (-111.4962, -128.4131)
  line L297 (-111.4962, -128.4131) -> (-113.4637, -124.9589)
  spline S144 degree 3 poles (-113.4637, -124.9589) (-114.535, -123.0788) (-116.2183, -120.1275) (-117.2239, -118.4223) knots 0 0 0 0 1 1 1 1
  line L298 (-117.2239, -118.4223) -> (-119.0385, -115.3398)
  line L299 (-119.0385, -115.3398) -> (-117.2239, -112.1918)
  spline S145 degree 3 poles (-117.2239, -112.1918) (-116.2183, -110.4647) (-114.535, -107.5571) (-113.4637, -105.7207) knots 0 0 0 0 1 1 1 1
  line L300 (-113.4637, -105.7207) -> (-111.5399, -102.3978)
  line L301 (-111.5399, -102.3978) -> (-103.9539, -102.3978)
  line L302 (-103.9539, -102.3978) -> (-96.3461, -102.3978)
  line L303 (-96.3461, -102.3978) -> (-93.5478, -107.251)
  spline S146 degree 3 poles (-37.91, -106.7045) (-36.5546, -109.0874) (-34.8712, -111.995) (-34.1935, -113.1755) knots 0 0 0 0 1 1 1 1
  line L304 (-34.1935, -113.1755) -> (-32.9255, -115.318)
  line L305 (-32.9255, -115.318) -> (-35.5927, -119.9526)
  spline S147 degree 3 poles (-35.5927, -119.9526) (-37.0792, -122.5104) (-38.7626, -125.4399) (-39.3747, -126.4893) knots 0 0 0 0 1 1 1 1
  line L306 (-39.3747, -126.4893) -> (-40.4459, -128.3912)
  line L307 (-40.4459, -128.3912) -> (-47.9882, -128.4131)
  line L308 (-47.9882, -128.4131) -> (-55.5305, -128.4131)
  line L309 (-55.5305, -128.4131) -> (-57.4324, -125.0683)
  spline S148 degree 3 poles (-57.4324, -125.0683) (-58.5036, -123.2537) (-60.187, -120.3024) (-61.2145, -118.5316) knots 0 0 0 0 1 1 1 1
  line L310 (-61.2145, -118.5316) -> (-63.0946, -115.318)
  line L311 (-63.0946, -115.318) -> (-60.9303, -111.6452)
  spline S149 degree 3 poles (-60.9303, -111.6452) (-59.7497, -109.634) (-58.0664, -106.7264) (-57.1919, -105.1742) knots 0 0 0 0 1 1 1 1
  line L312 (-57.1919, -105.1742) -> (-55.6179, -102.3978)
  line L313 (-55.6179, -102.3978) -> (-47.9882, -102.3978)
  line L314 (-47.9882, -102.3978) -> (-40.3804, -102.3978)
  line L315 (-40.3804, -102.3978) -> (-37.91, -106.7045)
  spline S150 degree 3 poles (-122.6456, -121.4611) (-121.6837, -123.1663) (-120.0004, -126.1176) (-118.8854, -128.0196) knots 0 0 0 0 1 1 1 1
  line L316 (-118.8854, -128.0196) -> (-116.8742, -131.4737)
  line L317 (-116.8742, -131.4737) -> (-120.5032, -137.748)
  spline S151 degree 3 poles (-120.5032, -137.748) (-122.4926, -141.224) (-124.2197, -144.1753) (-124.3508, -144.3283) knots 0 0 0 0 1 1 1 1
  spline S152 degree 3 poles (-124.3508, -144.3283) (-124.5039, -144.5251) (-126.2091, -144.5907) (-132.0243, -144.547) knots 0 0 0 0 1 1 1 1
  line L318 (-132.0243, -144.547) -> (-139.4791, -144.4814)
  line L319 (-139.4791, -144.4814) -> (-140.3754, -142.9511)
  spline S153 degree 3 poles (-140.3754, -142.9511) (-140.8564, -142.0985) (-142.5616, -139.1909) (-144.1575, -136.4582) knots 0 0 0 0 1 1 1 1
  line L320 (-144.1575, -136.4582) -> (-147.0213, -131.4956)
  line L321 (-147.0213, -131.4956) -> (-145.2068, -128.3694)
  spline S154 degree 3 poles (-145.2068, -128.3694) (-144.2012, -126.6423) (-142.5616, -123.8221) (-141.5559, -122.0732) knots 0 0 0 0 1 1 1 1
  spline S155 degree 3 poles (-141.5559, -122.0732) (-140.5722, -120.3243) (-139.654, -118.7721) (-139.5228, -118.6191) knots 0 0 0 0 1 1 1 1
  spline S156 degree 3 poles (-139.5228, -118.6191) (-139.3698, -118.4223) (-137.5771, -118.3567) (-131.8494, -118.3567) knots 0 0 0 0 1 1 1 1
  line L322 (-131.8494, -118.3567) -> (-124.3946, -118.3786)
  line L323 (-124.3946, -118.3786) -> (-122.6456, -121.4611)
  line L324 (-64.6905, -124.9808) -> (-60.9303, -131.4737)
  line L325 (-60.9303, -131.4737) -> (-63.2913, -135.5837)
  spline S157 degree 3 poles (-63.2913, -135.5837) (-64.5812, -137.8354) (-66.2645, -140.743) (-67.0297, -142.0766) knots 0 0 0 0 1 1 1 1
  line L326 (-67.0297, -142.0766) -> (-68.4288, -144.4814)
  line L327 (-68.4288, -144.4814) -> (-75.8836, -144.547)
  spline S158 degree 3 poles (-75.8836, -144.547) (-81.6988, -144.5907) (-83.404, -144.5251) (-83.5789, -144.3283) knots 0 0 0 0 1 1 1 1
  spline S159 degree 3 poles (-83.5789, -144.3283) (-83.6882, -144.1753) (-85.4153, -141.224) (-87.4047, -137.7699) knots 0 0 0 0 1 1 1 1
  line L328 (-87.4047, -137.7699) -> (-91.0337, -131.4956)
  line L329 (-91.0337, -131.4956) -> (-89.4815, -128.8066)
  spline S160 degree 3 poles (-89.4815, -128.8066) (-84.825, -120.7178) (-83.7538, -118.8814) (-83.5571, -118.6191) knots 0 0 0 0 1 1 1 1
  spline S161 degree 3 poles (-83.5571, -118.6191) (-83.3822, -118.4223) (-81.6988, -118.3567) (-75.9055, -118.4005) knots 0 0 0 0 1 1 1 1
  line L330 (-75.9055, -118.4005) -> (-68.4507, -118.466)
  line L331 (-68.4507, -118.466) -> (-64.6905, -124.9808)
  line L332 (-8.7247, -124.9808) -> (-4.9427, -131.4956)
  line L333 (-4.9427, -131.4956) -> (-8.4624, -137.5512)
  spline S162 degree 3 poles (-8.4624, -137.5512) (-10.3862, -140.8742) (-12.0696, -143.8255) (-12.2007, -144.1097) knots 0 0 0 0 1 1 1 1
  line L334 (-12.2007, -144.1097) -> (-12.4193, -144.5907)
  line L335 (-12.4193, -144.5907) -> (-19.9616, -144.547)
  line L336 (-19.9616, -144.547) -> (-27.5257, -144.4814)
  line L337 (-27.5257, -144.4814) -> (-28.422, -142.9511)
  spline S163 degree 3 poles (-28.422, -142.9511) (-28.9249, -142.0985) (-30.6301, -139.1909) (-32.2041, -136.4582) knots 0 0 0 0 1 1 1 1
  line L338 (-32.2041, -136.4582) -> (-35.068, -131.4956)
  line L339 (-35.068, -131.4956) -> (-31.4389, -125.1994)
  spline S164 degree 3 poles (-31.4389, -125.1994) (-29.4495, -121.7453) (-27.7225, -118.7721) (-27.5913, -118.6191) knots 0 0 0 0 1 1 1 1
  spline S165 degree 3 poles (-27.5913, -118.6191) (-27.4383, -118.4223) (-25.7331, -118.3567) (-19.9397, -118.4005) knots 0 0 0 0 1 1 1 1
  line L340 (-19.9397, -118.4005) -> (-12.4849, -118.466)
  line L341 (-12.4849, -118.466) -> (-8.7247, -124.9808)
extrude "Extrude6" cut sketch "Sketch6" against normal blind 70 contours S55 S56 S57 S58 S59 S60 L154 L155 L156 L157 S61 L158 L159 S62 L160 L161 L162 L163 | S63 L164 L165 S64 L166 L167 L168 L169 S65 L170 L171 S66 L172 L173 L174 L175 | S67 L176 L177 S68 L178 L179 L180 L181 S69 S70 S71 S72 L182 L183 L184 L185 | S73 S74 S75 L186 L187 L188 L189 S76 S77 L190 L191 L192 L193 | S78 S79 S80 S81 L194 L195 S82 S83 L196 L197 L198 L199 S84 L200 L201 L202 L203 | S85 S86 S87 S88 L204 L205 S89 S90 S91 S92 L206 L207 L208 L209 | S93 S94 S95 L210 L211 L212 L213 S96 L214 L215 L216 L217 L218 L219
